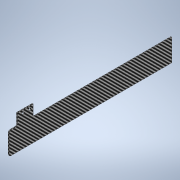
# Autodesk Inventor part: s_carbon_plate2
Saved by Autodesk Inventor 2022 (Build 260153000, 153)
## iProperties
Created: 2021-08-20
Part Number: s_carbon_plate2
Material: CFRP
Document SubType Name: Sheet Metal
Designer: yuta0
Density: 1.43 g/cm^3
Sheet Metal Rule: Default_mm
Appearance: カーボンファイバー
Author: yuta0
Autodesk Inventor part; units mm, degrees
ref_plane "YZ Plane" through (0, 0, 0) normal (1, 0, 0) x (0, 1, 0)
ref_plane "XZ Plane" through (0, 0, 0) normal (0, 1, 0) x (-1, 0, 0)
ref_plane "XY Plane" through (0, 0, 0) normal (0, 0, 1) x (1, 0, 0)
sketch "スケッチ1" plane through (0, 0, 0) normal (1, 0, 0) x (0, 1, 0)
  line L0 (-20.4, 93) -> (20.4, 93)
  line L1 (20.4, 93) -> (20.4, -93)
  line L2 (20.4, -93) -> (-20.4, -93)
  line L3 (-20.4, -93) -> (-20.4, 93)
  line L4 (-20.4, 93) -> (20.4, -93) construction
  line L5 (20.4, 93) -> (-20.4, -93) construction
  line L6 (20.4, 93) -> (-20.4, 93)
  line L7 (-20.4, 93) -> (-20.4, 95)
  line L8 (-20.4, 95) -> (20.4, 95)
  line L9 (20.4, 95) -> (20.4, 93)
  point P0 (0, 0)
  dimension "d0" = 40.8
  dimension "d1" = 186
  dimension "d19" = 2
  constraints: 20 end point, 4 parallel, 2 horizontal, 2 midpoint, 2 perpendicular
  measures "d0" distance of L0.start L0.end
  measures "d1" distance of L0.end L1.end
  measures "d19" distance between parallel lines of L0 L8
extrude "プレート1" add sketch "スケッチ1" along normal mid plane 1 contours L0 L1 L2 L3
sketch "スケッチ2" plane through (0.5, 0, 0) normal (1, 0, 0) x (0, 0, -1)
  line L0 (-93, 20.4) -> (93, 20.4) projected
  line L1 (-93, -20.4) -> (-93, 20.4) projected
  point P0 (0, 0)
  point P1 (-86, 16.4)
  point P2 (-78, 16.4)
  dimension "d3" = 4
  dimension "d4" = 7
  dimension "d5" = 8
  constraints: 1 horizontal alignment
  measures "d3" distance from line of L0 point (-86, 16.4)
  measures "d4" distance from line of L1 point (-86, 16.4)
  measures "d5" distance of point (-86, 16.4) point (-78, 16.4)
hole "穴1" at (0.5, 16.4, 86) at (0.5, 16.4, 78) direction (-1, 0, 0) diameter 3.2 end through all clearance for "Socket Head Cap Screw" size "M3" standard "Ansi Metric M Profile"
sketch "スケッチ3" plane through (-0.5, 0, 0) normal (-1, 0, 0) x (0, 0, 1)
  line L0 (-93, 20.4) -> (-93, -20.4) projected
  line L1 (-93, 20.4) -> (74, 20.4)
  line L2 (74, 20.4) -> (74, 6.6)
  line L3 (74, 6.6) -> (-93, 6.6)
  line L4 (-93, 6.6) -> (-93, 20.4)
  line L5 (-93, -20.4) -> (93, -20.4) projected
  line L6 (93, -20.4) -> (93, 20.4) projected
  point P0 (0, 0)
  point P1 (-93, 6.6)
  dimension "d14" = 19
  dimension "d18" = 13.8
  constraints: 8 end point, 2 parallel, 1 horizontal, 1 perpendicular
  measures "d14" distance between parallel lines of L6 L2
  measures "d18" distance between parallel lines of L3 L1
extrude "押し出し1" cut sketch "スケッチ3" against normal blind 10
sketch "スケッチ5" plane through (0.5, 0, 0) normal (1, 0, 0) x (0, 0, -1)
  line L0 (93, -20.4) -> (-93, -20.4)
  line L1 (-93, -20.4) -> (-103, -20.4)
  line L2 (-103, -20.4) -> (-103, 6.6)
  line L3 (-103, 6.6) -> (-93, 6.6)
  line L4 (-93, 6.6) -> (-93, -20.4)
  point P0 (0, 0)
  point P1 (-93, 20.4)
  dimension "d34" = 27
  dimension "d35" = 10
  measures "d34" distance of L1.end L2.end
  measures "d35" distance between parallel lines of L4 L2
sheet face with bend "面3" sketch "スケッチ5" thickness 1 toward (-1, 0, 0) bend radius 1 relief straight relief width 1 relief depth 0.5
bend "曲げ2"
fillet "コーナーR2" radius 2 4 edges at (0, 6.6, 74) (0, -20.4, 103) (0, 6.6, 103) (0, 6.6, 93)
equation "\"d11\" = Thickness"
equation "\"d2\" = Thickness"
equation "\"d28\" = BendRadius"
equation "\"d29\" = BendReliefWidth"
equation "\"d31\" = MinimumRemnant"
equation "\"d30\" = BendReliefDepth"
equation "\"d32\" = TransitionRadius"
equation "\"BendRadius\" = Thickness"
equation "\"BendReliefWidth\" = Thickness"
equation "\"BendReliefDepth\" = 0.5 * Thickness"
equation "\"CornerReliefSize\" = 4 * Thickness"
equation "\"MinimumRemnant\" = 2 * Thickness"
equation "\"TransitionRadius\" = BendRadius"
equation "\"JacobiRadiusSize\" = BendRadius"
equation "\"GapSize\" = Thickness"
equation "\"Thickness\" = 1"
